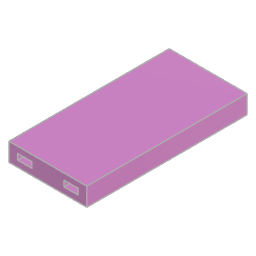
SBS_TTBB1000FASTA (Autodesk Fusion 360 design; units mm, degrees)
Autodesk Fusion 360 part; units mm, degrees
sketch "Sketch1" plane through (0, 0, 0) normal (0, 0, 1) x (1, 0, 0)
  line L0 (0, 0) -> (68, 0)
  line L1 (68, 0) -> (68, 140)
  line L2 (68, 140) -> (0, 140)
  line L3 (0, 140) -> (0, 0)
  dimension "d1" = 68
  dimension "d2" = 140
  constraint horizontal L0
  constraint vertical L1
  constraint horizontal L2
  constraint vertical L3
  constraint coincident L0.start L3.end
  measures "d1" distance of L0.start L0.end
  measures "d2" distance of L0.start L2.end
extrude "Extrude1" add sketch "Sketch1" along normal blind 16
sketch "Sketch2" plane through (0, 0, 0) normal (0, -1, 0) x (1, 0, 0)
  line L0 (0, 0) -> (68, 0)
  line L1 (68, 0) -> (68, 16)
  line L2 (68, 16) -> (0, 16)
  line L3 (0, 16) -> (0, 0)
  line L4 (0, 8) -> (68, 8) construction
  line L5 (7.5, 10.5) -> (20, 10.5)
  line L6 (20, 10.5) -> (20, 5.5)
  line L7 (20, 5.5) -> (7.5, 5.5)
  line L8 (7.5, 5.5) -> (7.5, 10.5)
  line L9 (7.5, 10.5) -> (20, 5.5) construction
  line L10 (20, 10.5) -> (7.5, 5.5) construction
  line L11 (34, 0) -> (34, 16) construction
  line L12 (60.5, 10.5) -> (48, 10.5)
  line L13 (60.5, 5.5) -> (60.5, 10.5)
  line L14 (48, 5.5) -> (60.5, 5.5)
  line L15 (48, 10.5) -> (48, 5.5)
  point P0 (13.75, 8)
  dimension "d5" = 12.5
  dimension "d6" = 5
  dimension "d7" = 7.5
  constraint midpoint L3 L4.start
  constraint midpoint L1 L4.end
  constraint horizontal L5
  constraint perpendicular L5 L6
  constraint parallel L5 L7
  constraint parallel L6 L8
  constraint coincident L9 P0
  constraint coincident L10 P0
  constraint coincident L4 P0
  constraint midpoint L0 L11.start
  constraint midpoint L2 L11.end
  constraint symmetric L5.start L11 L12.start
  constraint symmetric L5.end L11 L12.end
  constraint symmetric L6.end L11 L14.start
  constraint symmetric L7.end L11 L13.start
  measures "d5" distance of L6.end L7.end
  measures "d6" distance of L5.end L6.end
  measures "d7" distance of L3 L8
extrude "Extrude2" cut sketch "Sketch2" against normal blind 5 contours L5 L6 L7 L8 | L12 L13 L14 L15
named bodies: "powerbank"
